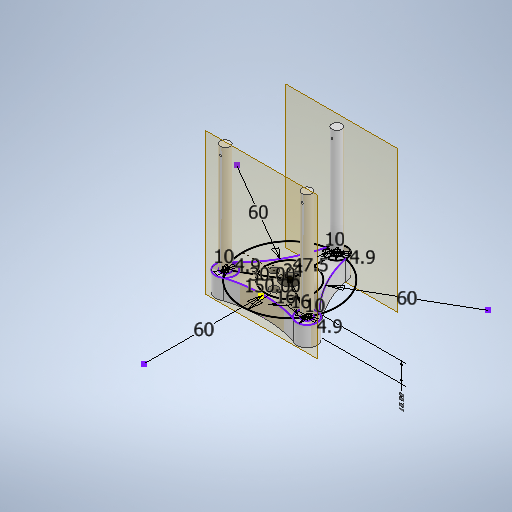
# Autodesk Inventor part: 바퀴연결
Saved by Autodesk Inventor 2025.1 (Build 291241000, 241)
## iProperties
Created: 2024-10-11
Part Number: 바퀴연결
Material: 일반
Document SubType Name: Sheet Metal
Designer: goode
Density: 1 g/cm^3
Sheet Metal Rule: 기본값_mm
Appearance: 기본값
Author: goode
Autodesk Inventor part; units mm, degrees
ref_plane "YZ Plane" through (0, 0, 0) normal (1, 0, 0) x (0, 1, 0)
ref_plane "XZ Plane" through (0, 0, 0) normal (0, 1, 0) x (-1, 0, 0)
sketch "스케치1" plane through (0, 0, 0) normal (0, 1, 0) x (-1, 0, 0)
  circle A0 centre (0, 0) radius 23.75
  line L0 (0, 0) -> (0, -23.75)
  line L1 (0, 0) -> (20.5681, 11.875)
  line L2 (0, 0) -> (23.75, 0) construction
  line L3 (0, 0) -> (-20.5681, 11.875)
  line L4 (0, 0) -> (23.75, 0) construction
  circle A1 centre (20.5681, 11.875) radius 5
  circle A2 centre (-20.5681, 11.875) radius 5
  circle A3 centre (0, -23.75) radius 5
  circle A4 centre (0, 0) radius 12
  arc A5 (-17.6262, 15.9179) -> (17.6262, 15.9179) centre (0, 73.2705) ccw
  arc A6 (22.5984, 7.3058) -> (4.9722, -23.2237) centre (63.4541, -36.6352) ccw
  arc A7 (-4.9722, -23.2237) -> (-22.5984, 7.3058) centre (-63.4541, -36.6352) ccw
  circle A8 centre (0, -23.75) radius 2.45
  circle A9 centre (-20.5681, 11.875) radius 2.45
  circle A10 centre (20.5681, 11.875) radius 2.45
  point P0 (-4.9722, -23.2237)
  dimension "d0" = 47.5
  dimension "d8" = 10
  dimension "d2" = 30
  dimension "d3" = 150
  dimension "d6" = 10
  dimension "d7" = 10
  dimension "d9" = 24
  dimension "d10" = 60
  dimension "d11" = 60
  dimension "d12" = 60
  dimension "d35" = 4.9
  dimension "d36" = 4.9
  dimension "d37" = 4.9
  constraints: 10 end point, 10 point on circle, 9 centre point, 6 coincident, 2 equal length, 2 horizontal, 1 vertical, 14 other
  measures "d2" angle of L2 L1
  measures "d3" angle of L4 L3
  measures "d6" diameter of A1
  measures "d7" diameter of A2
  measures "d9" diameter of A4
  measures "d10" radius of A5
  measures "d11" radius of A6
  measures "d12" radius of A7
  measures "d35" diameter of A8
  measures "d36" diameter of A9
  measures "d37" diameter of A10
sketch "스케치2" plane through (0, 0, 0) normal (0, 1, 0) x (-1, 0, 0)
  point P0 (0, 0)
extrude "돌출3" add sketch "스케치1" against normal blind 5 contours A1 L1 A10 A0 | A0 A10 A1 | A6 A3 L0 A4 L1 A1 | A3 A0 A8 | A0 A8 L0 A3 | A10 L1 A0 | A0 A10 | A1 A0 A10 L1 | L1 A4 L3 A2 A5 A1 | A8 A0 | A0 L0 A8 | A3 A7 A2 L3 A4 L0 | L0 A8 A0 A3 | L1 A10 A0 | A4 L0 L1 | L1 L3 A4 | A0 A8 L0 | A4 L3 L0 | A2 L3 A9 A0 | A0 A9 A2 | A0 A9 L3 A2 | A9 L3 A0 | A0 A9 | A0 L3 A9
sketch "스케치3" plane through (0, -5, 0) normal (0, -1, 0) x (1, 0, 0)
  point P0 (0, 0)
extrude "돌출4" add sketch "스케치1" against normal blind 10 contours A1 L1 A10 A0 | A0 A10 A1 | A6 A3 L0 A4 L1 A1 | A3 A0 A8 | A0 A8 L0 A3 | A10 L1 A0 | A0 A10 | A1 A0 A10 L1 | L1 A4 L3 A2 A5 A1 | A8 A0 | A0 L0 A8 | A3 A7 A2 L3 A4 L0 | L0 A8 A0 A3 | L1 A10 A0 | A4 L0 L1 | L1 L3 A4 | A0 A8 L0 | A4 L3 L0 | A2 L3 A9 A0 | A0 A9 A2 | A0 A9 L3 A2 | A9 L3 A0 | A0 A9 | A0 L3 A9
sketch "스케치4" plane through (0, -10, 0) normal (0, -1, 0) x (1, 0, 0)
  circle A0 centre (0, 0) radius 8
  circle A1 centre (0, 0) radius 8
  point P0 (8, 0)
  point P1 (0, -8)
  point P2 (0, 8)
  point P3 (-8, 0)
  point P4 (-8, 0)
  point P5 (-8, 0)
  point P6 (0, 8)
  point P7 (8, 0)
  point P8 (0, -8)
  dimension "d24" = 16
  dimension "d26" = 16
  constraints: 7 point on circle, 4 coincident, 2 centre point
  measures "d24" diameter of A0
  measures "d26" diameter of A1
sketch "스케치5" plane through (0, 0, 0) normal (0, 1, 0) x (1, 0, 0)
  circle A0 centre (0, 0) radius 8
  point P0 (8, 0)
  point P1 (0, -8)
  point P2 (-8, 0)
  point P3 (0, 8)
  dimension "d27" = 16
  constraints: 4 point on circle, 1 centre point, 1 coincident
  measures "d27" diameter of A0
hole "구멍1" at (0, 0, 8) at (-8, 0, 0) at (0, 0, -8) at (8, 0, 0) direction (0, -1, 0) diameter 2.2 end through all counterbore diameter 4.2 counterbore depth 7
sketch "스케치6" plane through (0, 0, 0) normal (0, 1, 0) x (1, 0, 0)
  point P0 (0, 0)
sketch "스케치7" plane through (0, 0, 0) normal (0, 1, 0) x (1, 0, 0)
  point P0 (0, 0)
extrude "돌출6" add sketch "스케치1" along normal blind 55 contours A10 L1 A0 | A0 A10 | A8 A0 | A0 L0 A8 | L1 A10 A0 | A0 A8 L0 | A9 L3 A0 | A0 A9 | A0 L3 A9
sketch "스케치8" plane through (0, 0, 0) normal (0, 1, 0) x (1, 0, 0)
  circle A0 centre (0, 0) radius 4.5
  dimension "d40" = 9
  constraints: 1 centre point, 1 coincident
  measures "d40" diameter of A0
extrude "돌출7" cut sketch "스케치8" against normal blind 55
sketch "스케치9" plane through (0, 0, 0) normal (1, 0, 0) x (0, 1, 0)
  point P0 (0, 0)
ref_plane "작업 평면1" through (0, 0, -26.2) normal (0, 0, 1) x (1, 0, 0)
ref_plane "작업 평면2" through (-20.5681, 0, 14.325) normal (0, 0, 1) x (1, 0, 0)
sketch "스케치10" plane through (0, 0, -26.2) normal (0, 0, 1) x (1, 0, 0)
  line L0 (2.45, 55) -> (-2.45, 55) projected
  line L1 (0, 55) -> (0, 51)
  circle A0 centre (0, 51) radius 0.5
  point P0 (0, 0)
  dimension "d43" = 4
  dimension "d48" = 1
  constraints: 2 end point, 1 centre point, 1 coincident, 1 midpoint, 1 vertical
  measures "d43" distance of L1.start L1.end
  measures "d48" diameter of A0
sketch "스케치11" plane through (-20.5681, 0, 14.325) normal (0, 0, 1) x (1, 0, 0)
  point P0 (20.5681, 0)
sketch "스케치12" plane through (-20.5681, 0, 14.325) normal (0, 0, 1) x (1, 0, 0)
  line L0 (2.45, 55) -> (-2.45, 55) projected
  line L1 (0, 55) -> (0, 51)
  circle A0 centre (0, 51) radius 0.5
  line L2 (43.5862, 55) -> (38.6862, 55) projected
  line L3 (41.1362, 55) -> (41.1362, 51)
  circle A1 centre (41.1362, 51) radius 0.5
  point P0 (20.5681, 0)
  dimension "d44" = 4
  dimension "d45" = 1
  dimension "d46" = 4
  dimension "d47" = 1
  constraints: 4 end point, 2 centre point, 2 coincident, 2 midpoint, 2 vertical
  measures "d44" distance of L1.start L1.end
  measures "d45" diameter of A0
  measures "d46" distance of L3.start L3.end
  measures "d47" diameter of A1
extrude "돌출8" cut sketch "스케치10" along normal up to next
extrude "돌출9" cut sketch "스케치12" against normal up to surface (40.525 mm away)
equation "\"d19\" = d7"
equation "\"TransitionRadius\" = BendRadius"
equation "\"BendRadius\" = 0.5"
